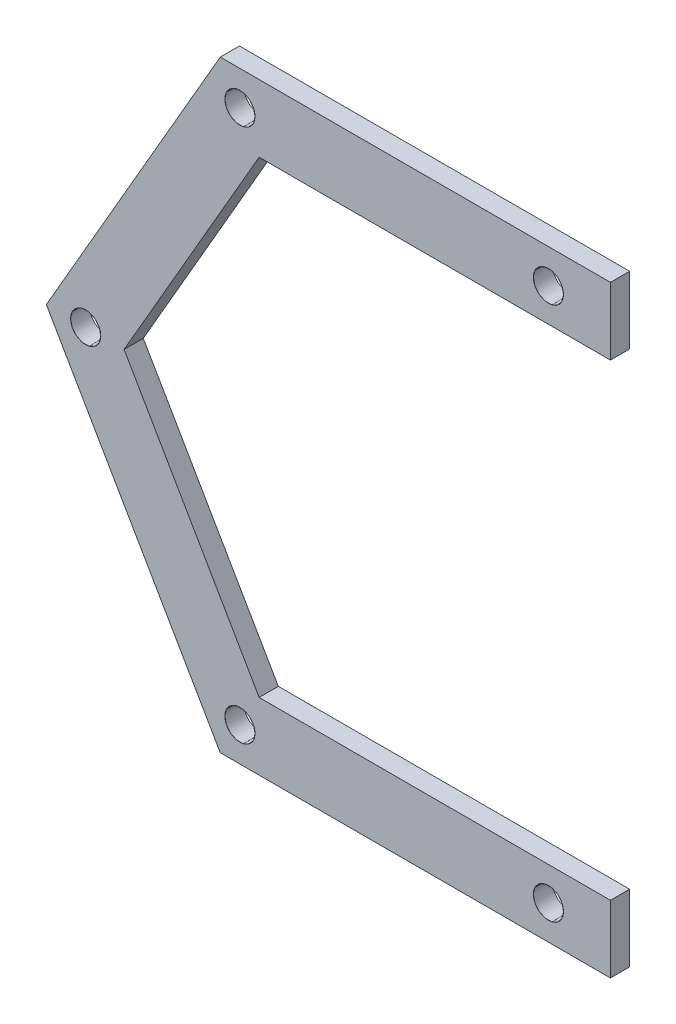
# Autodesk Inventor part: AW01
Saved by Autodesk Inventor 2017 (Build 210142000, 142)
## iProperties
Created: 2019-07-25
Part Number: AW01
Material: Stainless Steel
Document SubType Name: Modeling
Designer: Dell
Density: 8 g/cm^3
Appearance: Semi-Polished
Author: Dell
Autodesk Inventor part; units mm, degrees
ref_plane "YZ Plane" through (0, 0, 0) normal (1, 0, 0) x (0, 1, 0)
ref_plane "XZ Plane" through (0, 0, 0) normal (0, 1, 0) x (-1, 0, 0)
ref_plane "XY Plane" through (0, 0, 0) normal (0, 0, 1) x (1, 0, 0)
sketch "Sketch1" plane through (0, 0, 0) normal (0, 0, 1) x (1, 0, 0)
  circle A0 centre (-10.2528, 5.6292) radius 2.5
  circle A1 centre (-61.2528, 93.9638) radius 2.5
  circle A2 centre (-10.2528, 93.9638) radius 2.5
  circle A3 centre (-86.7528, 49.7965) radius 2.5
  circle A4 centre (-61.2528, 5.6292) radius 2.5
  line L0 (0, 0) -> (-64.5028, 0)
  line L1 (0, 0) -> (0, 12.1292)
  line L2 (0, 12.1292) -> (-57.5, 12.1292)
  line L3 (-57.5, 12.1292) -> (-79.2472, 49.7965)
  line L4 (-79.2472, 49.7965) -> (-57.5, 87.4638)
  line L5 (-57.5, 87.4638) -> (0, 87.4638)
  line L6 (0, 87.4638) -> (0, 99.5929)
  line L7 (-64.5028, 99.5929) -> (0, 99.5929)
  line L8 (-93.2528, 49.7965) -> (-64.5028, 99.5929)
  line L9 (-64.5028, 0) -> (-93.2528, 49.7965)
  dimension "d0" = 75.3346
  dimension "d1" = 99.5929
  dimension "d2" = 57.5
  dimension "d3" = 12.1292
  dimension "d4" = 120
  dimension "d5" = 120
  dimension "d6" = 12.1292
  dimension "d7" = 12.1292
  dimension "d8" = 10.2528
  dimension "d9" = 3.25
  dimension "d10" = 6.5
  dimension "d11" = 5.6292
  dimension "d12" = 5.6292
  dimension "d13" = 10.2528
  dimension "d14" = 3.25
  dimension "d15" = 5.6292
  dimension "d16" = 5
  dimension "d17" = 5
  dimension "d18" = 5
  dimension "d19" = 5
  dimension "d20" = 5
  constraints: 20 end point, 5 centre point, 3 perpendicular, 3 vertical alignment, 2 horizontal alignment, 2 parallel, 1 coincident
  measures "d0" distance between parallel lines of L2 L5
  measures "d1" distance between parallel lines of L0 L7
  measures "d2" distance of L4.end L5.end
  measures "d3" distance of L0.start L1.end
  measures "d4" angle of L5 L4
  measures "d5" angle of L2 L3
  measures "d6" distance between parallel lines of L9 L3
  measures "d7" distance between parallel lines of L8 L4
  measures "d8" distance from line of L1 A0.centre
  measures "d9" horizontal distance of L0.end A4.centre
  measures "d10" distance of L8.start A3.centre
  measures "d11" distance from line of L7 A1.centre
  measures "d12" distance from line of L7 A2.centre
  measures "d13" distance from line of L6 A2.centre
  measures "d14" horizontal distance of L7.start A1.centre
  measures "d15" distance from line of L0 A4.centre
  measures "d16" diameter of A0
  measures "d17" diameter of A4
  measures "d18" diameter of A3
  measures "d19" diameter of A1
  measures "d20" diameter of A2
extrude "Extrusion1" add sketch "Sketch1" along normal blind 3.175
sketch "Sketch2" plane through (0, 0, 3.175) normal (0, 0, 1) x (1, 0, 0)
  line L0 (-57.5, 87.4638) -> (0, 87.4638) projected
  line L1 (-79.2472, 49.7965) -> (-57.5, 87.4638) projected
  line L2 (-57.5, 12.1292) -> (-79.2472, 49.7965) projected
  line L3 (0, 12.1292) -> (-57.5, 12.1292) projected
  line L4 (0, 88.4638) -> (-58.0774, 88.4638)
  line L5 (-58.0774, 88.4638) -> (-80.4019, 49.7965)
  line L6 (-80.4019, 49.7965) -> (-58.0774, 11.1292)
  line L7 (-58.0774, 11.1292) -> (0, 11.1292)
  line L8 (0, 87.4638) -> (0, 88.4638)
  line L9 (0, 87.4638) -> (0, 99.5929) projected
  line L10 (0, 0) -> (0, 12.1292) projected
  line L11 (0, 11.1292) -> (0, 12.1292)
  dimension "d23" = 1
  constraints: 12 end point, 1 collinear, 3 other
  measures "d23" distance between parallel lines of L0 L4
extrude "Extrusion2" cut sketch "Sketch2" against normal through all
equation "\"d6\" = d3"
equation "\"d7\" = d3"
body "Solid1"
